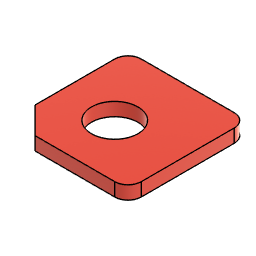
sample assemble project (Autodesk Fusion 360 archive; units mm, degrees)
design "ex 1"
part number: 2025-08-27-18-34-59-648
part number: 2025-08-27-18-35-13-303
Autodesk Fusion 360 part; units mm, degrees
sketch "Sketch1" plane through (0, 0, 0) normal (0, 0, 1) x (1, 0, 0) in component "base"
  line L0 (0, 0) -> (80, 0)
  line L1 (90, 10) -> (90, 80)
  line L2 (80, 90) -> (10, 90)
  line L3 (0, 80) -> (0, 0)
  line L4 (0, 20) -> (20, 0)
  line L5 (0, 20) -> (25.31, 20) construction
  circle A0 centre (40, 40) radius 17.5
  arc A1 (10, 90) -> (0, 80) centre (10, 80) ccw
  arc A2 (90, 80) -> (80, 90) centre (80, 80) ccw
  arc A3 (80, 0) -> (90, 10) centre (80, 10) ccw
  point P0 (90, 0)
  point P1 (0, 90)
  dimension "d1" = 90
  dimension "d2" = 90
  dimension "d3" = 45
  dimension "d4" = 20
  dimension "d5" = 20
  dimension "d6" = 35
  dimension "d7" = 40
  dimension "d8" = 40
  dimension "d9" = 10
  dimension "d10" = 10
  dimension "d11" = 10
  constraint horizontal L0
  constraint vertical L1
  constraint horizontal L2
  constraint vertical L3
  constraint coincident L0.start L3.end
  constraint horizontal L5
  constraint coincident L3 L4.start
  constraint coincident L0 L4.end
  constraint coincident P1 L3
  constraint coincident P1 L2
  constraint tangent L3 A1
  constraint tangent L2 A1
  constraint tangent L2 A2
  constraint tangent L1 A2
  constraint coincident P0 L0
  constraint coincident P0 L1
  constraint tangent L0 A3
  constraint tangent L1 A3
  measures "d1" distance of L0.start P0
  measures "d2" distance of L0.start P1
  measures "d3" angle of L4 L5
  measures "d4" distance of L0.start L4.start
  measures "d5" distance of L0.start L4.end
  measures "d6" diameter of A0
  measures "d7" distance of L3 A0.centre
  measures "d8" distance of L0 A0.centre
  measures "d9" radius of A1
  measures "d10" radius of A2
  measures "d11" radius of A3
extrude "Extrude1" add sketch "Sketch1" along normal blind 10 contours L0 L1 L2 L3 L4 A1 A2 A3 in component "base"
component "base" placed x (1, 0, 0) y (0, 1, 0) z (0, 0, 1) at (0, 0, 0)

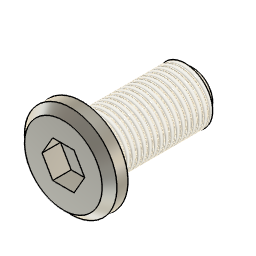
design "screw"
part number: 2025-08-27-19-08-21-093
Autodesk Fusion 360 part; units mm, degrees
sketch "Sketch1" plane through (0, 0, 0) normal (0, 1, 0) x (1, 0, 0)
  circle A0 centre (0, 0) radius 7.5
  dimension "d1" = 15
  constraint coincident A0.centre origin
  measures "d1" diameter of A0
extrude "Extrude1" add sketch "Sketch1" along normal blind 30
sketch "Sketch2" plane through (0, 0, 0) normal (0, -1, 0) x (1, 0, 0)
  circle A0 centre (0, 0) radius 7.5
  circle A1 centre (0, 0) radius 12.5
  dimension "d4" = 25
  constraint concentric A0 A1
  measures "d4" diameter of A1
extrude "Extrude2" add sketch "Sketch2" along normal blind 5 contours A0 | A1
chamfer "Chamfer1" distance 2 angle 45 2 edges at (-11.6541, -5, -4.5202) (-6.9925, 30, 2.7121)
thread "Thread1" "ISO Metric profile 15.0 M15x1.5 M15x1.5 6g" major diameter 14.85 minor diameter 13.1369 pitch 1.5 angle 60 resizes the face on face at (7.4907, 18.6667, 0.3738)
sketch "Sketch3" plane through (0, -5, 0) normal (0, -1, 0) x (1, 0, 0)
  circle A0 centre (0, 0) radius 10.5
  line L0 (5.7735, 0) -> (2.8868, 5)
  line L1 (2.8868, 5) -> (-2.8868, 5)
  line L2 (-2.8868, 5) -> (-5.7735, 0)
  line L3 (-5.7735, 0) -> (-2.8868, -5)
  line L4 (-2.8868, -5) -> (2.8868, -5)
  line L5 (2.8868, -5) -> (5.7735, 0)
  dimension "d10" = 5
  constraint coincident A0.centre origin
  constraint horizontal L1
  measures "d10" distance of A0.centre L5
extrude "Extrude3" cut sketch "Sketch3" against normal blind 5 contours L0 L1 L2 L3 L4 L5

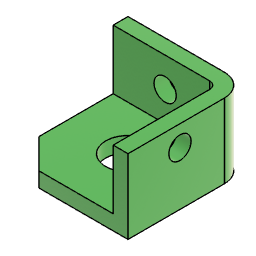
design "ex1.2"
part number: 2025-08-27-18-51-06-745
part number: 2025-08-27-18-51-33-151
Autodesk Fusion 360 part; units mm, degrees
sketch "Sketch1" plane through (0, 0, 0) normal (0, 0, 1) x (1, 0, 0) in component "side"
  line L0 (0, 0) -> (80, 0)
  line L1 (80, 0) -> (80, 80)
  line L2 (80, 80) -> (0, 80)
  line L3 (0, 80) -> (0, 0)
  line L4 (0, 20) -> (20, 0)
  line L5 (0, 20) -> (22.9559, 20) construction
  circle A0 centre (40, 40) radius 15
  dimension "d1" = 80
  dimension "d2" = 80
  dimension "d3" = 45
  dimension "d4" = 20
  dimension "d5" = 20
  dimension "d6" = 30
  dimension "d7" = 40
  dimension "d8" = 40
  constraint horizontal L0
  constraint vertical L1
  constraint horizontal L2
  constraint vertical L3
  constraint coincident L0.start L3.end
  constraint horizontal L5
  constraint coincident L3 L4.start
  measures "d1" distance of L0.start L0.end
  measures "d2" distance of L0.start L2.end
  measures "d3" angle of L4 L5
  measures "d4" horizontal distance of L0.start L4.end
  measures "d5" distance of L0.start L4.start
  measures "d6" diameter of A0
  measures "d7" distance of L3 A0.centre
  measures "d8" distance of L0 A0.centre
extrude "Extrude1" add sketch "Sketch1" along normal blind 10 contours L0 L1 L2 L3 L4 in component "side"
sketch "Sketch2" plane through (0, 0, 10) normal (0, 0, 1) x (-1, 0, 0) in component "side"
  circle A0 centre (-40, -40) radius 15
  line L0 (0, -20) -> (-20, 0)
  line L1 (-20, 0) -> (-80, 0)
  line L2 (-80, 0) -> (-80, -80)
  line L3 (-80, -80) -> (0, -80)
  line L4 (0, -80) -> (0, -20)
  line L5 (0, -80) -> (-80, -80)
  line L6 (-80, -80) -> (-80, -70)
  line L7 (-80, -70) -> (0, -70)
  line L8 (0, -70) -> (0, -80)
  line L9 (-80, -80) -> (-70, -80)
  line L10 (-70, -80) -> (-70, 0)
  line L11 (-70, 0) -> (-80, 0)
  line L12 (-80, 0) -> (-80, -80)
  dimension "d11" = 10
  dimension "d12" = 10
  constraint horizontal L5
  constraint vertical L6
  constraint horizontal L7
  constraint vertical L8
  constraint coincident L3.end L4.start
  constraint horizontal L9
  constraint vertical L10
  constraint horizontal L11
  constraint vertical L12
  constraint coincident L2.end L3.start
  measures "d11" distance of L5 L7
  measures "d12" distance of L10 L12
extrude "Extrude2" add sketch "Sketch2" along normal blind 40 contours L3 L4 L5 L7 L8 L10 | L1 L2 L7 L10 L11 L12 | L2 L3 L5 L6 L7 L9 L10 L12 in component "side"
fillet "Fillet1" radius 5 1 edges at (70, 70, 30) in component "side"
fillet "Fillet2" radius 15 1 edges at (80, 80, 25) in component "side"
sketch "Sketch3" plane through (70, 0, 0) normal (-1, 0, 0) x (0, -1, 0) in component "side"
  line L0 (-65, 50) -> (-65, 10)
  line L1 (-65, 10) -> (0, 10)
  line L2 (0, 10) -> (0, 50)
  line L3 (0, 50) -> (-65, 50)
  circle A0 centre (-35, 36.0439) radius 7.5
  dimension "d19" = 15
  dimension "d20" = 35
  dimension "d21" = 26.0439
  measures "d19" diameter of A0
  measures "d20" distance of L2 A0.centre
  measures "d21" distance of L1 A0.centre
extrude "Extrude3" cut sketch "Sketch3" against normal blind 10 contours A0 in component "side"
sketch "Sketch4" plane through (0, 70, 0) normal (0, -1, 0) x (1, 0, 0) in component "side"
  line L0 (65, 10) -> (65, 50)
  line L1 (65, 50) -> (0, 50)
  line L2 (0, 50) -> (0, 10)
  line L3 (0, 10) -> (65, 10)
  circle A0 centre (35, 30) radius 7.5
  dimension "d24" = 15
  dimension "d25" = 35
  dimension "d26" = 20
  measures "d24" diameter of A0
  measures "d25" distance of L2 A0.centre
  measures "d26" distance of L3 A0.centre
extrude "Extrude4" cut sketch "Sketch4" against normal blind 10 contours A0 in component "side"
component "side" placed x (1, 0, 0) y (0, 1, 0) z (0, 0, 1) at (0, 0, 0)
